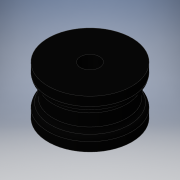
# Autodesk Inventor part: Pulley
Saved by Autodesk Inventor 2016 (Build 200138000, 138)
## iProperties
Created: 2015-11-23
Part Number: Pulley
Material: Acetal Resin, Black
Document SubType Name: Modeling
Designer: Julia
Density: 1.425 g/cm^3
Appearance: Smooth - Black
Author: Julia
Autodesk Inventor part; units mm, degrees
ref_plane "YZ Plane" through (0, 0, 0) normal (1, 0, 0) x (0, 1, 0)
ref_plane "XZ Plane" through (0, 0, 0) normal (0, 1, 0) x (-1, 0, 0)
ref_plane "XY Plane" through (0, 0, 0) normal (0, 0, 1) x (1, 0, 0)
sketch "Sketch1" plane through (0, 0, 0) normal (0, 1, 0) x (-1, 0, 0)
  circle A0 centre (0, 0) radius 87.757
  dimension "d0" = 175.514
  constraints: 1 centre point, 1 coincident
  measures "d0" diameter of A0
extrude "Extrusion1" add sketch "Sketch1" along normal blind 54.61
sketch "Sketch2" plane through (0, 54.61, 0) normal (0, 1, 0) x (1, 0, 0)
  circle A0 centre (0, 0) radius 99.949
  dimension "d3" = 199.898
  constraints: 1 centre point, 1 coincident
  measures "d3" diameter of A0
sketch "Sketch3" plane through (0, 0, 0) normal (0, -1, 0) x (1, 0, 0)
  circle A0 centre (0, 0) radius 99.949
  dimension "d4" = 199.898
  constraints: 1 centre point, 1 coincident
  measures "d4" diameter of A0
extrude "Extrusion2" add sketch "Sketch2" along normal blind 30.48
extrude "Extrusion3" add sketch "Sketch3" along normal blind 30.48
sketch "Sketch4" plane through (0, 85.09, 0) normal (0, 1, 0) x (1, 0, 0)
  circle A0 centre (0, 0) radius 22.86
  dimension "d9" = 45.72
  constraints: 1 centre point, 1 coincident
  measures "d9" diameter of A0
extrude "Extrusion4" cut sketch "Sketch4" against normal blind 115.57
fillet "Fillet1" radius 12.7 1 edges at (87.757, 54.61, 0)
fillet "Fillet2" radius 12.7 1 edges at (87.757, 0, 0)
fillet "Fillet3" radius 12.7 4 edges at (0, 0, 99.949) (0, 0, -99.949) (0, 54.5998, 99.949) (0, 54.5998, -99.949)
body "Solid1"
